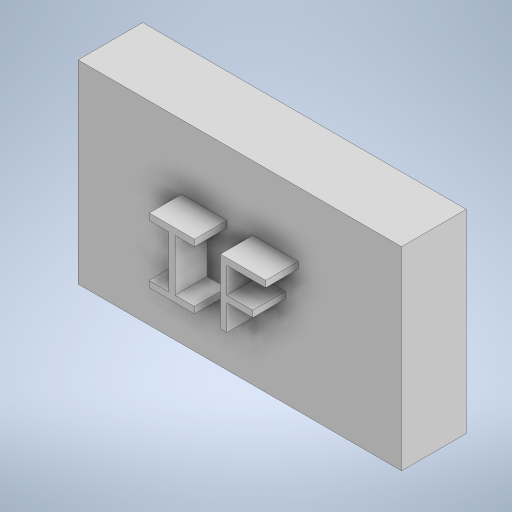
# Autodesk Inventor part: Names
Saved by Autodesk Inventor 2023.1 (Build 271208000, 208)
## iProperties
Created: 2022-08-24
Part Number: Names
Material: Generic
Document SubType Name: Modeling
Designer: felip
Density: 1 g/cm^3
Appearance: Default
Author: felip
Autodesk Inventor part; units mm, degrees
ref_plane "YZ Plane" through (0, 0, 0) normal (1, 0, 0) x (0, 1, 0)
ref_plane "XZ Plane" through (0, 0, 0) normal (0, 1, 0) x (-1, 0, 0)
ref_plane "XY Plane" through (0, 0, 0) normal (0, 0, 1) x (1, 0, 0)
sketch "Sketch1" plane through (0, 0, 0) normal (0, 0, 1) x (1, 0, 0)
  line L0 (0, 0) -> (50, 0)
  line L1 (50, 0) -> (50, 30)
  line L2 (50, 30) -> (0, 30)
  line L3 (0, 30) -> (0, 0)
  dimension "d0" = 50
  dimension "d1" = 30
  constraints: 8 end point, 2 parallel, 1 horizontal, 1 perpendicular
  measures "d0" distance of L1.end L2.end
  measures "d1" distance of L0.end L1.end
extrude "Extrusion1" add sketch "Sketch1" along normal blind 10
sketch "Sketch2" plane through (0, 0, 10) normal (0, 0, 1) x (1, 0, 0)
  line L0 (0, 0) -> (50, 0) projected
  line L1 (50, 30) -> (0, 30) projected
  line L2 (0, 0) -> (50, 0)
  line L3 (50, 0) -> (50, 30)
  line L4 (50, 30) -> (0, 30)
  line L5 (0, 30) -> (0, 0)
  line L6 (16, 20) -> (23, 20)
  line L7 (23, 20) -> (23, 19)
  line L8 (23, 19) -> (20, 19)
  line L9 (20, 19) -> (20, 11)
  line L10 (20, 11) -> (23, 11)
  line L11 (23, 11) -> (23, 10)
  line L12 (23, 10) -> (16, 10)
  line L13 (16, 10) -> (16, 11)
  line L14 (16, 11) -> (19, 11)
  line L15 (19, 11) -> (19, 19)
  line L16 (19, 19) -> (16, 19)
  line L17 (16, 19) -> (16, 20)
  line L18 (27, 10) -> (27, 20)
  line L19 (27, 20) -> (34, 20)
  line L20 (34, 20) -> (34, 19)
  line L21 (34, 19) -> (28, 19)
  line L22 (28, 19) -> (28, 15)
  line L23 (28, 15) -> (32, 15)
  line L24 (32, 15) -> (32, 14)
  line L25 (32, 14) -> (28, 14)
  line L26 (28, 14) -> (28, 10)
  line L27 (28, 10) -> (27, 10)
  point P0 (17.5, 19)
  point P1 (16, 10.5)
  point P2 (23, 10.5)
  point P3 (23, 19.5)
  point P4 (31, 19)
  point P5 (30, 14)
  point P6 (27, 15)
  dimension "d4" = 1
  dimension "d5" = 1
  dimension "d6" = 1
  dimension "d7" = 3
  dimension "d8" = 3
  dimension "d9" = 10
  dimension "d10" = 10
  dimension "d11" = 30
  dimension "d12" = 50
  dimension "d13" = 23
  dimension "d14" = 23
  dimension "d15" = 10
  dimension "d16" = 1
  dimension "d17" = 1
  dimension "d18" = 1
  dimension "d19" = 7
  dimension "d20" = 4
  dimension "d21" = 10
  dimension "d22" = 4
  constraints: 52 end point, 17 perpendicular, 9 point on line, 7 midpoint, 2 horizontal, 2 parallel, 1 vertical
  measures "d4" distance from line of point (17.5, 19) L6
  measures "d5" distance between parallel lines of L9 L15
  measures "d6" distance between parallel lines of L12 L14
  measures "d7" distance from line of point (16, 10.5) L15
  measures "d8" distance from line of point (23, 10.5) L9
  measures "d9" distance between parallel lines of L12 L6
  measures "d10" distance between parallel lines of L6 L1
  measures "d11" distance of L4.end L0.start
  measures "d12" distance of L0.start L0.end
  measures "d13" distance from line of point (23, 19.5) L5
  measures "d14" distance between parallel lines of L3 L18
  measures "d15" distance between parallel lines of L1 L19
  measures "d16" distance from line of point (31, 19) L19
  measures "d17" distance from line of point (30, 14) L23
  measures "d18" distance from line of point (27, 15) L22
  measures "d19" distance of L18.end L19.end
  measures "d20" distance of L22.end L23.end
  measures "d21" distance between parallel lines of L27 L19
  measures "d22" distance between parallel lines of L23 L21
extrude "Extrusion2" add sketch "Sketch2" along normal blind 5 contours L6 L7 L8 L9 L10 L11 L12 L13 L14 L15 L16 L17 | L18 L19 L20 L21 L22 L23 L24 L25 L26 L27
equation "\"d4\" = d5"
equation "\"d6\" = d5"
equation "\"d8\" = d7"
equation "\"d10\" = -0.5 * d9 + 0.5 * d11"
equation "\"d14\" = d13"
equation "\"d15\" = d10"
equation "\"d16\" = d5"
equation "\"d17\" = d5"
equation "\"d18\" = d5"
equation "\"d19\" = d8 + d7 + d5"
equation "\"d20\" = d7 + d5"
equation "\"d21\" = d9"
equation "\"d22\" = -0.5 * d17 + 0.5 * d21 - 0.5 * d16"
body "Solid1"
